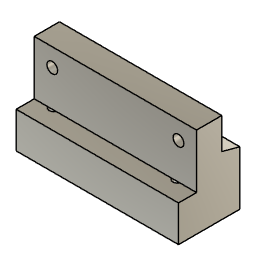
Filamentschrank Magnethalterung Tür (Autodesk Fusion 360 design; units mm, degrees)
Autodesk Fusion 360 part; units mm, degrees
sketch "Skizze1" plane through (0, 0, 0) normal (0, 0, 1) x (1, 0, 0)
  line L0 (0, 0) -> (45, 0)
  line L1 (45, 0) -> (45, 17)
  line L2 (45, 17) -> (0, 17)
  line L3 (0, 17) -> (0, 0)
  line L4 (0, 0) -> (45, 0)
  line L5 (45, 0) -> (45, 5)
  line L6 (45, 5) -> (0, 5)
  line L7 (0, 5) -> (0, 0)
  line L8 (45, 17) -> (0, 17)
  line L9 (0, 17) -> (0, 12)
  line L10 (0, 12) -> (45, 12)
  line L11 (45, 12) -> (45, 17)
  line L12 (45, 0) -> (39.2, 0)
  line L13 (39.2, 0) -> (39.2, 5.5)
  line L14 (39.2, 5.5) -> (45, 5.5)
  line L15 (45, 5.5) -> (45, 0)
  line L16 (0, 0) -> (4.9, 0)
  line L17 (4.9, 0) -> (4.9, 5.5)
  line L18 (4.9, 5.5) -> (0, 5.5)
  line L19 (0, 5.5) -> (0, 0)
  dimension "d1" = 45
  dimension "d2" = 17
  dimension "d3" = 5
  dimension "d8" = 5
  dimension "d12" = 5.8
  dimension "d13" = 5.5
  dimension "d14" = 4.9
  dimension "d15" = 5.5
  constraint horizontal L0
  constraint vertical L1
  constraint horizontal L2
  constraint vertical L3
  constraint coincident L0.start L3.end
  constraint horizontal L4
  constraint vertical L5
  constraint horizontal L6
  constraint vertical L7
  constraint horizontal L8
  constraint vertical L9
  constraint horizontal L10
  constraint vertical L11
  constraint horizontal L12
  constraint vertical L13
  constraint horizontal L14
  constraint vertical L15
  constraint horizontal L16
  constraint vertical L17
  constraint horizontal L18
  constraint vertical L19
  measures "d1" distance of L0.start L0.end
  measures "d2" distance of L0.start L2.end
  measures "d3" distance of L0.start L6.end
  measures "d8" distance of L1.end L10.end
  measures "d12" distance of L0.end L12.end
  measures "d13" distance of L0.end L14.end
  measures "d14" distance of L0.start L16.end
  measures "d15" distance of L0.start L18.end
extrude "Extrusion1" add sketch "Skizze1" along normal blind 25 contours L3 L6 L17 L18 L19 | L1 L3 L6 L10 L13 L14 L17 L18 | L1 L6 L13 L14 L15 | L1 L2 L3 L8 L9 L10 L11
extrude "Extrusion2" add sketch "Skizze1" along normal blind 10 contours L0 L3 L4 L6 L7 L16 L17 L19 | L0 L4 L6 L13 L17 | L0 L1 L4 L5 L6 L12 L13 L15
extrude "Extrusion3" cut sketch "Skizze1" along normal blind 10 from surface at 15 contours L1 L2 L3 L8 L9 L10 L11
sketch "Skizze2" plane through (0, 12, 0) normal (0, 1, 0) x (-1, 0, 0)
  line L0 (-45, 15) -> (0, 15)
  line L1 (0, 15) -> (0, 25)
  line L2 (0, 25) -> (-45, 25)
  line L3 (-45, 25) -> (-45, 15)
  line L4 (0, 25) -> (-5, 25)
  line L5 (-5, 25) -> (-5, 20)
  line L6 (-5, 20) -> (0, 20)
  line L7 (0, 20) -> (0, 25)
  line L8 (-45, 25) -> (-40, 25)
  line L9 (-40, 25) -> (-40, 20)
  line L10 (-40, 20) -> (-45, 20)
  line L11 (-45, 20) -> (-45, 25)
  dimension "d19" = 5
  dimension "d20" = 5
  dimension "d21" = 5
  dimension "d22" = 5
  constraint horizontal L4
  constraint vertical L5
  constraint horizontal L6
  constraint vertical L7
  constraint coincident L1.end L2.start
  constraint horizontal L8
  constraint vertical L9
  constraint horizontal L10
  constraint vertical L11
  constraint coincident L2.end L3.start
  measures "d19" distance of L1.end L4.end
  measures "d20" distance of L1.end L6.end
  measures "d21" distance of L2.end L8.end
  measures "d22" distance of L2.end L10.end
draft "Verjüngung1" angle 15 neutral plane through (45, 17, 0) pull (0, 1, 0) 1 faces at (15, 15.3333, 15)
hole "Bohrung3" at (39.2, 5.5, 0) at (4.9, 5.5, 0) direction (0, 0, 1) diameter 2.5 depth 10 tip angle 180
hole "Bohrung4" at (40, 12, 20) at (5, 12, 20) direction (0, -1, 0) diameter 3 depth 10 tip angle 180 countersink diameter 6.5 countersink angle 90
